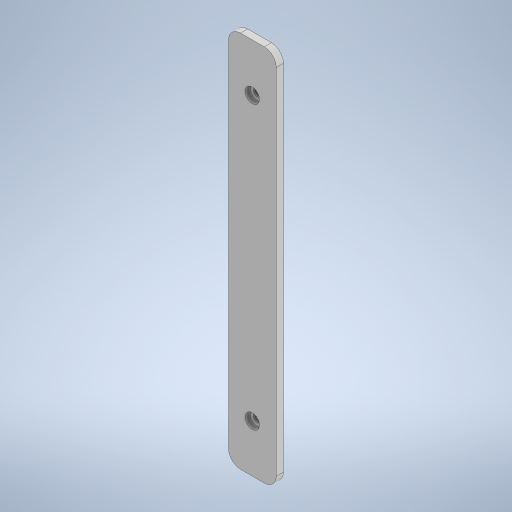
# Autodesk Inventor part: BP_BOX-Bar
Saved by Autodesk Inventor 2024.3 (Build 283343000, 343)
## iProperties
Created: 2025-10-31
Part Number: BP_BOX-Bar
Material: 一般
Document SubType Name: Modeling
Designer: 佐藤智貴
Density: 1 g/cm^3
Appearance: 既定
Author: 佐藤智貴
Autodesk Inventor part; units mm, degrees
ref_plane "YZ Plane" through (0, 0, 0) normal (1, 0, 0) x (0, 1, 0)
ref_plane "XZ Plane" through (0, 0, 0) normal (0, 1, 0) x (-1, 0, 0)
ref_plane "XY Plane" through (0, 0, 0) normal (0, 0, 1) x (1, 0, 0)
sketch "スケッチ1" plane through (0, 0, 0) normal (0, 0, 1) x (1, 0, 0)
  line L0 (0, 0) -> (20, 0)
  line L1 (20, 0) -> (20, 158)
  line L2 (20, 158) -> (0, 158)
  line L3 (0, 158) -> (0, 0)
  dimension "d0" = 158
  dimension "d1" = 20
  constraints: 8 end point, 2 parallel, 1 horizontal, 1 perpendicular
  measures "d0" distance of L0.end L1.end
  measures "d1" distance of L1.end L2.end
extrude "押し出し1" add sketch "スケッチ1" along normal blind 3
sketch "スケッチ2" plane through (0, 0, 3) normal (0, 0, 1) x (1, 0, 0)
  line L0 (0, 0) -> (20, 0) projected
  line L1 (20, 0) -> (20, 158) projected
  point P0 (10, 138)
  point P1 (10, 20)
  dimension "d4" = 20
  dimension "d5" = 118
  dimension "d6" = 10
  dimension "d7" = 10
  measures "d4" distance from line of L0 point (10, 20)
  measures "d5" distance of point (10, 20) point (10, 138)
  measures "d6" distance from line of L1 point (10, 138)
  measures "d7" distance from line of L1 point (10, 20)
hole "穴1" at (10, 138, 3) at (10, 20, 3) direction (0, 0, -1) diameter 3.2 depth 8
sketch "スケッチ3" plane through (0, 0, 3) normal (0, 0, 1) x (1, 0, 0)
  circle A0 centre (10, 20) radius 1.6 projected
  circle A1 centre (10, 138) radius 1.6 projected
  line L0 (20, 0) -> (20, 158) projected
  line L1 (20, 158) -> (0, 158) projected
  line L2 (0, 158) -> (0, 0) projected
  line L3 (0, 0) -> (20, 0) projected
  circle A2 centre (10, 138) radius 3
  circle A3 centre (10, 20) radius 3
  dimension "d15" = 6
  dimension "d16" = 6
  constraints: 2 centre point
  measures "d15" diameter of A3
  measures "d16" diameter of A2
extrude "押し出し2" cut sketch "スケッチ3" against normal blind 2 contours A1 | A2 | A3
fillet "フィレット1" radius 5 4 edges at (0, 158, 1.5) (20, 158, 1.5) (0, 0, 1.5) (20, 0, 1.5)
equation "\"d7\" = d6"
equation "\"d16\" = d15"
